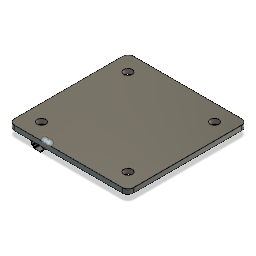
Distribution board v1 (Autodesk Fusion 360 design; units mm, degrees)
Autodesk Fusion 360 part; units mm, degrees
sketch "Sketch1" plane through (0, 0, 0) normal (0, 1, 0) x (1, 0, 0)
  line L0 (21.0617, -21.0617) -> (-21.0617, -21.0617)
  line L1 (-21.0617, -21.0617) -> (-21.0617, 21.0617)
  line L2 (-21.0617, 21.0617) -> (21.0617, 21.0617)
  line L3 (21.0617, 21.0617) -> (21.0617, -21.0617)
  line L4 (21.0617, -21.0617) -> (-21.0617, 21.0617) construction
  line L5 (-21.0617, -21.0617) -> (21.0617, 21.0617) construction
  line L6 (15.25, -15.25) -> (-15.25, -15.25) construction
  line L7 (-15.25, -15.25) -> (-15.25, 15.25) construction
  line L8 (-15.25, 15.25) -> (15.25, 15.25) construction
  line L9 (15.25, 15.25) -> (15.25, -15.25) construction
  line L10 (15.25, -15.25) -> (-15.25, 15.25) construction
  line L11 (-15.25, -15.25) -> (15.25, 15.25) construction
  constraint horizontal L0
  constraint perpendicular L0 L1
  constraint parallel L0 L2
  constraint parallel L1 L3
  constraint coincident L4 origin
  constraint coincident L5 origin
  constraint equal L2 L3
  constraint horizontal L6
  constraint perpendicular L6 L7
  constraint parallel L6 L8
  constraint parallel L7 L9
  constraint coincident L10 origin
  constraint coincident L11 origin
  constraint equal L8 L9
sketch "Sketch2" plane through (0, 0, 0) normal (0, 1, 0) x (1, 0, 0)
  circle A0 centre (-15.25, 15.25) radius 1.5
  circle A1 centre (15.25, 15.25) radius 1.5
  circle A2 centre (15.25, -15.25) radius 1.5
  circle A3 centre (-15.25, -15.25) radius 1.5
  point P0 (-15.25, 15.25)
  point P1 (15.25, 15.25)
  point P2 (15.25, -15.25)
  point P3 (-15.25, -15.25)
  constraint coincident P0 A0.centre
  constraint coincident P1 A1.centre
  constraint coincident P2 A2.centre
  constraint coincident P3 A3.centre
extrude "Extrude1" add sketch "Sketch1" along normal blind 1.75 makes body 1
hole "Hole1" at (15.25, 0, 15.25) at (-15.25, 0, 15.25) at (-15.25, 0, -15.25) at (15.25, 0, -15.25) direction (0, 1, 0) diameter 3 end through all bodies 1
fillet "Fillet1" radius 2 1 edges at (-21.0617, 0.875, -21.0617) on bodies 1
fillet "Fillet2" radius 2 1 edges at (21.0617, 0.875, -21.0617) on bodies 1
fillet "Fillet3" radius 2 1 edges at (21.0617, 0.875, 21.0617) on bodies 1
fillet "Fillet4" radius 2 1 edges at (-21.0617, 0.875, 21.0617) on bodies 1
sketch "Sketch3" plane through (0, 0, 0) normal (0, 0, 1) x (1, 0, 0)
sketch "Sketch4" plane through (0, 0, 0) normal (0, 0, 1) x (1, 0, 0)
  line L0 (-8.9, 0, 21) -> (-13, 0, 21)
  line L1 (-13, 0, 21) -> (-13, -1.2, 21)
  line L2 (-12.1219, -2, 21) -> (-9.7796, -2, 21)
  line L3 (-8.9, -1.1, 21) -> (-8.9, 0, 21)
  line L4 (-9.5796, -1.8, 21) -> (-9.5796, -1.5, 21)
  line L5 (-9.3796, -1.3, 21) -> (-9.1, -1.3, 21)
  line L6 (-12.8, -1.4, 21) -> (-12.5219, -1.4, 21)
  line L7 (-12.3219, -1.6, 21) -> (-12.3219, -1.8, 21)
  arc A0 through (-9.1, -1.3, 21) (-8.9586, -1.2414, 21) (-8.9, -1.1, 21)
  arc A1 through (-9.3796, -1.3, 21) (-9.521, -1.3586, 21) (-9.5796, -1.5, 21)
  arc A2 through (-9.7796, -2, 21) (-9.6381, -1.9414, 21) (-9.5796, -1.8, 21)
  arc A3 through (-12.3219, -1.8, 21) (-12.2633, -1.9414, 21) (-12.1219, -2, 21)
  arc A4 through (-12.3219, -1.6, 21) (-12.3805, -1.4586, 21) (-12.5219, -1.4, 21)
  arc A5 through (-13, -1.2, 21) (-12.9414, -1.3414, 21) (-12.8, -1.4, 21)
  line L8 (-12.9, -0.1, 21) -> (-12.9, -1.2, 21)
  arc A6 through (-12.9, -1.2, 21) (-12.8707, -1.2707, 21) (-12.8, -1.3, 21)
  line L9 (-12.8, -1.3, 21) -> (-12.5219, -1.3, 21)
  arc A7 through (-12.2219, -1.6, 21) (-12.3098, -1.3879, 21) (-12.5219, -1.3, 21)
  line L10 (-12.2219, -1.6, 21) -> (-12.2219, -1.8, 21)
  arc A8 through (-12.2219, -1.8, 21) (-12.1926, -1.8707, 21) (-12.1219, -1.9, 21)
  line L11 (-12.1219, -1.9, 21) -> (-9.7796, -1.9, 21)
  arc A9 through (-9.7796, -1.9, 21) (-9.7088, -1.8707, 21) (-9.6796, -1.8, 21)
  line L12 (-9.6796, -1.8, 21) -> (-9.6796, -1.5, 21)
  arc A10 through (-9.3796, -1.2, 21) (-9.5917, -1.2879, 21) (-9.6796, -1.5, 21)
  line L13 (-9.3796, -1.2, 21) -> (-9.1, -1.2, 21)
  arc A11 through (-9.1, -1.2, 21) (-9.0293, -1.1707, 21) (-9, -1.1, 21)
  line L14 (-9, -1.1, 21) -> (-9, -0.1, 21)
  line L15 (-9, -0.1, 21) -> (-12.9, -0.1, 21)
sketch "Sketch5" plane through (0, 0, 21.0617) normal (0, 0, 1) x (1, 0, 0)
  line L0 (-19.0617, 1.75) -> (-19.0617, 0)
  line L1 (-19.0617, 0) -> (19.0617, 0)
  line L2 (19.0617, 0) -> (19.0617, 1.75)
  line L3 (19.0617, 1.75) -> (-19.0617, 1.75)
extrude "Extrude2" add sketch "Sketch4" against normal blind 3 contours L0 L1 L2 L3 L4 L5 L6 L7 A0 A1 A2 A3 A4 A5 in plane through (0, 0, 21) normal (0, 0, 1) bodies 1
sketch "Sketch6" plane through (0, 0, 0) normal (1, 0, 0) x (0, 0, -1)
sketch "Sketch7" plane through (0, 0, 18) normal (0, 0, -1) x (-1, 0, 0)
  line L0 (9.3796, -1.2) -> (9.1, -1.2)
  arc A0 (9, -1.1) -> (9.1, -1.2) centre (9.1, -1.1) ccw
  line L1 (9, -1.1) -> (9, -0.1)
  line L2 (9, -0.1) -> (12.9, -0.1)
  line L3 (12.9, -0.1) -> (12.9, -1.2)
  arc A1 (12.8, -1.3) -> (12.9, -1.2) centre (12.8, -1.2) ccw
  line L4 (12.8, -1.3) -> (12.5219, -1.3)
  arc A2 (12.5219, -1.3) -> (12.2219, -1.6) centre (12.5219, -1.6) ccw
  line L5 (12.2219, -1.6) -> (12.2219, -1.8)
  arc A3 (12.1219, -1.9) -> (12.2219, -1.8) centre (12.1219, -1.8) ccw
  line L6 (12.1219, -1.9) -> (9.7796, -1.9)
  arc A4 (9.6796, -1.8) -> (9.7796, -1.9) centre (9.7796, -1.8) ccw
  line L7 (9.6796, -1.8) -> (9.6796, -1.5)
  arc A5 (9.6796, -1.5) -> (9.3796, -1.2) centre (9.3796, -1.5) ccw
  line L8 (9.1, -1.3) -> (9.3796, -1.3)
  arc A6 (9.5796, -1.5) -> (9.3796, -1.3) centre (9.3796, -1.5) ccw
  line L9 (9.5796, -1.5) -> (9.5796, -1.8)
  arc A7 (9.5796, -1.8) -> (9.7796, -2) centre (9.7796, -1.8) ccw
  line L10 (9.7796, -2) -> (12.1219, -2)
  arc A8 (12.1219, -2) -> (12.3219, -1.8) centre (12.1219, -1.8) ccw
  line L11 (12.3219, -1.8) -> (12.3219, -1.6)
  arc A9 (12.5219, -1.4) -> (12.3219, -1.6) centre (12.5219, -1.6) ccw
  line L12 (12.5219, -1.4) -> (12.8, -1.4)
  arc A10 (12.8, -1.4) -> (13, -1.2) centre (12.8, -1.2) ccw
  line L13 (13, -1.2) -> (13, 0)
  line L14 (13, 0) -> (8.9, 0)
  line L15 (8.9, 0) -> (8.9, -1.1)
  arc A11 (8.9, -1.1) -> (9.1, -1.3) centre (9.1, -1.1) ccw
  line L16 (13, 0) -> (13, -1.2)
  line L17 (12.8, -1.4) -> (12.5219, -1.4)
  line L18 (12.3219, -1.6) -> (12.3219, -1.8)
  line L19 (12.1219, -2) -> (9.7796, -2)
  line L20 (9.5796, -1.8) -> (9.5796, -1.5)
  line L21 (9.3796, -1.3) -> (9.1, -1.3)
  line L22 (8.9, -1.1) -> (8.9, 0)
  constraint coincident L13.end L14.start
  constraint coincident A10.end L13.start
  constraint coincident L12.end A10.start
  constraint coincident A9.start L12.start
  constraint coincident L11.end A9.end
  constraint coincident A8.end L11.start
  constraint coincident L10.end A8.start
  constraint coincident A7.end L10.start
  constraint coincident L9.end A7.start
  constraint coincident A6.start L9.start
  constraint coincident L8.end A6.end
  constraint coincident L8.start A11.end
  constraint coincident L15.end A11.start
  constraint coincident L14.end L15.start
extrude "Extrude3" add sketch "Sketch7" along normal blind 0.5 separate body contours L0 A0 L1 L2 L3 A1 L4 A2 L5 A3 L6 A4 L7 A5 makes body 2
sketch "Sketch8" plane through (0, 0, 17.5) normal (0, 0, -1) x (-1, 0, 0)
  arc A0 (9.6796, -1.8) -> (9.7796, -1.9) centre (9.7796, -1.8) ccw
  line L0 (9.7796, -1.9) -> (12.1219, -1.9)
  arc A1 (12.1219, -1.9) -> (12.2219, -1.8) centre (12.1219, -1.8) ccw
  line L1 (12.2219, -1.8) -> (12.2219, -1.6)
  arc A2 (12.5219, -1.3) -> (12.2219, -1.6) centre (12.5219, -1.6) ccw
  line L2 (12.5219, -1.3) -> (12.8, -1.3)
  arc A3 (12.8, -1.3) -> (12.9, -1.2) centre (12.8, -1.2) ccw
  line L3 (12.9, -1.2) -> (12.9, -0.1)
  line L4 (12.9, -0.1) -> (9, -0.1)
  line L5 (9, -0.1) -> (9, -1.1)
  arc A4 (9, -1.1) -> (9.1, -1.2) centre (9.1, -1.1) ccw
  line L6 (9.1, -1.2) -> (9.3796, -1.2)
  arc A5 (9.6796, -1.5) -> (9.3796, -1.2) centre (9.3796, -1.5) ccw
  line L7 (9.6796, -1.5) -> (9.6796, -1.8)
  circle A6 centre (11, -1) radius 0.3086
  circle A7 centre (11.858, -1) radius 0.3086
  circle A8 centre (10.1696, -1) radius 0.3086
  constraint equal A6 A8
  constraint equal A6 A7
